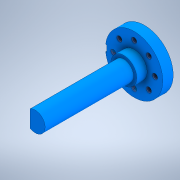
# Autodesk Inventor part: BM-MX28
Saved by Autodesk Inventor 2021 (Build 250183000, 183)
## iProperties
Created: 2022-05-03
Part Number: BM-MX28
Material: PETG
Document SubType Name: Modeling
Designer: Alcatraz
Density: 1.27 g/cm^3
Appearance: Genérico
Author: Alcatraz
Autodesk Inventor part; units mm, degrees
ref_plane "XY Plane" through (0, 0, 0) normal (0, 0, 1) x (1, 0, 0)
sketch "Boceto1" plane through (0, 0, 0) normal (0, 0, 1) x (1, 0, 0)
  circle A0 centre (0, 0) radius 11
  dimension "d0" = 22
  constraints: 1 centre point, 1 coincident
  measures "d0" diameter of A0
extrude "Extrusión1" add sketch "Boceto1" along normal blind 4
sketch "Boceto2" plane through (0, 0, 4) normal (0, 0, 1) x (1, 0, 0)
  line L0 (0, 0) -> (0, 8)
  circle A0 centre (0, 8) radius 1
  dimension "d3" = 8
  dimension "d4" = 2
  constraints: 2 end point, 1 centre point, 1 coincident, 1 vertical
  measures "d3" distance of L0.start L0.end
  measures "d4" diameter of A0
hole "Agujero1" at (0, 8, 4) direction (0, 0, -1) diameter 2.013 end through all thread size "M2.5x0.45" class "6H" standard "ISO Metric profile"
pattern_circular "Patrón circular1" count 8 over 360 about axis through (0, 0, 0) along (0, 0, 1) of "Agujero1"
sketch "Boceto3" plane through (0, 0, 0) normal (0, 0, -1) x (-1, 0, 0)
  circle A0 centre (0, 0) radius 4.4
  dimension "d15" = 8.8
  constraints: 1 centre point, 1 coincident
  measures "d15" diameter of A0
extrude "Extrusión2" cut sketch "Boceto3" against normal blind 2.9
sketch "Boceto4" plane through (0, 0, 2.9) normal (0, 0, -1) x (-1, 0, 0)
  circle A0 centre (0, 0) radius 2.5
  dimension "d18" = 5
  constraints: 1 centre point, 1 coincident
  measures "d18" diameter of A0
extrude "Extrusión3" cut sketch "Boceto4" against normal blind 2.6
sketch "Boceto5" plane through (0, 0, 4) normal (0, 0, 1) x (1, 0, 0)
  circle A0 centre (0, 0) radius 5
  dimension "d21" = 10
  constraints: 1 centre point, 1 coincident
  measures "d21" diameter of A0
extrude "Extrusión4" add sketch "Boceto5" along normal blind 4
sketch "Boceto6" plane through (0, 0, 8) normal (0, 0, 1) x (1, 0, 0)
  arc A0 (-1.9, -3.2909) -> (-1.9, 3.2909) centre (0, 0) ccw
  line L0 (0, 0) -> (-1.9, 0)
  line L1 (-1.9, 0) -> (-1.9, 3.2909)
  line L2 (-1.9, 0) -> (-1.9, -3.2909)
  dimension "DiametroEje" = 7.6
  dimension "d26" = 1.9
  constraints: 6 end point, 2 point on circle, 1 centre point, 1 coincident, 1 horizontal, 1 point on line, 1 vertical
  measures "DiametroEje" diameter of A0
  measures "d26" distance of L0.start L0.end
extrude "Extrusión5" add sketch "Boceto6" along normal blind 34
ref_plane "Plano de trabajo1" through (0, 11, 0) normal (0, 1, 0) x (-1, 0, 0)
ref_plane "Plano de trabajo2" through (-11, 0, 0) normal (1, 0, 0) x (0, 1, 0)
sketch "Boceto8" plane through (-11, 0, 0) normal (1, 0, 0) x (0, 1, 0)
  line L0 (-1.25, 0) -> (1.25, 0)
  line L1 (1.25, 0) -> (1.25, 4)
  line L2 (1.25, 4) -> (-1.25, 4)
  line L3 (-1.25, 4) -> (-1.25, 0)
  line L4 (-1.25, 0) -> (1.25, 4) construction
  line L5 (1.25, 0) -> (-1.25, 4) construction
  point P0 (0, 0)
  point P1 (0, 2)
  dimension "d33" = 2.5
  dimension "d34" = 4
  constraints: 12 end point, 2 midpoint, 2 parallel, 1 horizontal, 1 perpendicular
  measures "d33" distance of L2.end L1.end
  measures "d34" distance of L1.end L0.end
extrude "Extrusión7" cut sketch "Boceto8" along normal blind 0.5
equation "\"d26\" = 0.25 * DiametroEje"
